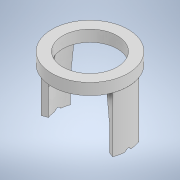
# Autodesk Inventor part: cable_jig_holder
Saved by Autodesk Inventor 2022 (Build 260153000, 153)
## iProperties
Created: 2022-03-09
Part Number: cable_jig_holder
Material: Generic
Document SubType Name: Modeling
Designer: kylem
Density: 1 g/cm^3
Appearance: Default
Author: kylem
Autodesk Inventor part; units mm, degrees
ref_plane "YZ Plane" through (0, 0, 0) normal (1, 0, 0) x (0, 1, 0)
ref_plane "XZ Plane" through (0, 0, 0) normal (0, 1, 0) x (-1, 0, 0)
ref_plane "XY Plane" through (0, 0, 0) normal (0, 0, 1) x (1, 0, 0)
sketch "Sketch1" plane through (0, 0, 0) normal (0, 1, 0) x (-1, 0, 0)
  circle A0 centre (0, 0) radius 35
  circle A1 centre (0, 0) radius 29.75
  dimension "d0" = 70
  dimension "d1" = 59.5
  constraints: 2 centre point, 2 coincident
  measures "d0" diameter of A0
  measures "d1" diameter of A1
extrude "Extrusion1" add sketch "Sketch1" along normal blind 10.5
sketch "Sketch2" plane through (0, 0, 0) normal (0, -1, 0) x (1, 0, 0)
  line L0 (0, 0) -> (37.5877, -13.6808)
  line L1 (0, 0) -> (40, 0) construction
  line L2 (0, 0) -> (6.8145, 0)
  circle A0 centre (0, 0) radius 29.75
  circle A1 centre (0, 0) radius 34.95
  line L3 (0, 0) -> (37.5877, 13.6808)
  line L4 (0, 0) -> (0, 5.9562)
  line L5 (0, 0) -> (-37.5877, -13.6808)
  line L6 (0, 0) -> (-37.5877, 13.6808)
  point P0 (-32.8423, -11.9536)
  point P1 (-27.9559, -10.1751)
  point P2 (-27.9559, 10.1751)
  point P3 (-32.8423, 11.9536)
  point P4 (32.8423, 11.9536)
  point P5 (27.9559, 10.1751)
  point P6 (27.9559, -10.1751)
  point P7 (32.8423, -11.9536)
  dimension "d4" = 40
  dimension "d5" = 20
  constraints: 14 end point, 3 symmetric about line, 2 centre point, 2 coincident, 1 equal length, 1 horizontal, 1 point on line, 1 vertical
  measures "d4" distance of L0.start L0.end
  measures "d5" angle of L0 L1
extrude "Extrusion2" add sketch "Sketch2" along normal blind 51 contours A0 L3 A1 L0 | L5 A1 L6 A0
sketch "Sketch3" plane through (0, -51, 0) normal (0, -1, 0) x (1, 0, 0)
  arc A0 (-27.9559, 10.1751) -> (-27.9559, -10.1751) centre (0, 0) ccw projected
  circle A1 centre (0, 0) radius 29.75
  arc A2 (-32.8423, 11.9536) -> (-32.8423, -11.9536) centre (0, 0) ccw projected
  circle A3 centre (0, 0) radius 34.95
  line L0 (0, 0) -> (38.637, 10.3528)
  line L1 (0, 0) -> (40, 0) construction
  line L2 (0, 0) -> (-5.4085, 0)
  line L3 (-5.4085, 0) -> (0, 0)
  line L4 (0, 0) -> (0, 7.8245)
  line L5 (0, 0) -> (38.637, -10.3528)
  line L6 (0, 0) -> (-38.637, -10.3528)
  line L7 (0, 0) -> (-33.7591, 9.0457)
  line L8 (-33.7591, 9.0457) -> (-28.7363, 7.6999)
  line L9 (-28.7363, -7.6999) -> (-33.7591, -9.0457)
  circle A4 centre (-31.2477, 8.3728) radius 1.4
  circle A5 centre (-31.2477, -8.3728) radius 1.4
  circle A6 centre (31.2477, 8.3728) radius 1.4
  circle A7 centre (31.2477, -8.3728) radius 1.4
  point P0 (-38.637, 10.3528)
  dimension "d8" = 40
  dimension "d9" = 15
  dimension "d10" = 2.8
  constraints: 20 end point, 6 centre point, 6 point on circle, 6 symmetric about line, 4 point on line, 2 coincident, 1 collinear, 1 equal length, 1 horizontal, 1 midpoint, 1 vertical, 3 other
  measures "d8" distance of L0.start L0.end
  measures "d9" angle of L1 L0
  measures "d10" diameter of A4
extrude "Extrusion3" cut sketch "Sketch3" against normal blind 15 contours A4 L7 | L7 A4 | A6 L0 | L0 A6 | A5 L6 | L6 A5 | A7 L5 | L5 A7
sketch "Sketch4" plane through (0, 0, 0) normal (1, 0, 0) x (0, 1, 0)
  line L0 (-51, 11.9536) -> (-51, -11.9536) projected
  line L1 (-51, 0) -> (-52.5, 0)
  circle A0 centre (-52.5, 0) radius 3.25
  line L2 (-49.25, 0) -> (-48.75, 0)
  line L3 (-48.75, 0) -> (-49.6833, 1.6214)
  line L4 (-48.75, 0) -> (-49.6833, -1.6214)
  point P0 (0, 0)
  point P1 (-51, 2.8831)
  point P2 (-51, -2.8831)
  dimension "d13" = 1.5
  dimension "d14" = 6.5
  dimension "d15" = 0.5
  constraints: 8 end point, 3 point on circle, 2 tangent, 1 centre point, 1 coincident, 1 horizontal, 1 midpoint, 1 perpendicular
  measures "d13" distance of L1.start L1.end
  measures "d14" diameter of A0
  measures "d15" distance of L2.start L2.end
extrude "Extrusion4" cut sketch "Sketch4" along normal mid plane 1500 contours A0 L0 | L3 L2 A0 | L2 L4 A0 picked at (-50.8278, 1.8106)
sketch "Sketch6" plane through (0, 10.5, 0) normal (0, 1, 0) x (1, 0, 0)
  circle A0 centre (0, 0) radius 29.75
  circle A1 centre (0, 0) radius 25
  dimension "d30" = 50
  constraints: 2 centre point, 2 coincident
  measures "d30" diameter of A1
extrude "Extrusion6" add sketch "Sketch6" against normal blind 10.5
chamfer "Chamfer2" distance 26.93 angle 10 1 edges at (-29.75, 0, 0) measured on face at (-29.75, -0.5, 0)
chamfer "Chamfer3" distance 26.93 angle 10 1 edges at (29.75, 0, 0) measured on face at (29.75, -0.5, 0)
body "Solid1"
